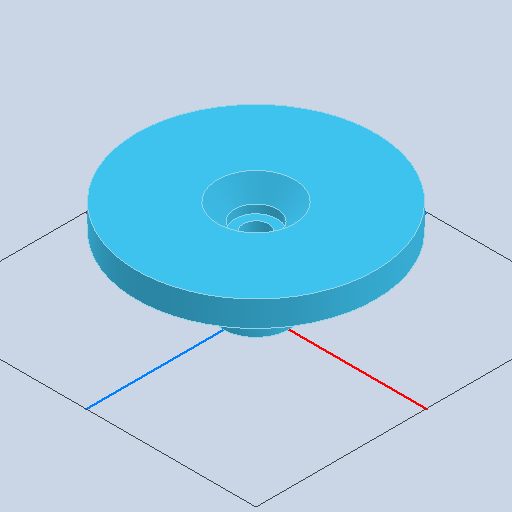
# Autodesk Inventor part: 000.005.002.003 - ВТУЛКА
Saved by Autodesk Inventor 2022 (Build 260153000, 153)
## iProperties
Created: 2022-11-19
Part Number: 000.005.002.003 - ВТУЛКА
Material: Пластик АБС
Document SubType Name: Modeling
Designer: Petrov Ivan
Density: 1.06 g/cm^3
Appearance: Бирюзовый
Mass: 2.20089 g
Surface Area: 17.8832 cm^2
Volume: 2.07631 cm^3
Author: Petrov Ivan
Autodesk Inventor part; units mm, degrees
ref_plane "YZ Plane" through (0, 0, 0) normal (1, 0, 0) x (0, 1, 0)
ref_plane "XZ Plane" through (0, 0, 0) normal (0, 1, 0) x (-1, 0, 0)
ref_plane "XY Plane" through (0, 0, 0) normal (0, 0, 1) x (1, 0, 0)
sketch "Эскиз1" plane through (0, 0, 0) normal (0, 1, 0) x (-1, 0, 0)
  circle A0 centre (0, 0) radius 3.9
  dimension "d0" = 7.8
  constraints: 1 centre point, 1 coincident
  measures "d0" diameter of A0
extrude "Выдавливание1" add sketch "Эскиз1" along normal blind 8.05
sketch "Эскиз2" plane through (0, 8.05, 0) normal (0, 1, 0) x (1, 0, 0)
  circle A0 centre (0, 0) radius 1.5
  dimension "d3" = 3
  constraints: 1 centre point, 1 coincident
  measures "d3" diameter of A0
extrude "Выдавливание2" cut sketch "Эскиз2" against normal blind 8.05
sketch "Эскиз3" plane through (0, 8.05, 0) normal (0, 1, 0) x (1, 0, 0)
  circle A0 centre (0, 0) radius 14
  circle A1 centre (0, 0) radius 1.5 projected
  dimension "d6" = 28
  constraints: 1 centre point, 1 coincident
  measures "d6" diameter of A0
extrude "Выдавливание3" add sketch "Эскиз3" along normal blind 3
sketch "Эскиз4" plane through (0, 11.05, 0) normal (0, 1, 0) x (1, 0, 0)
  circle A0 centre (0, 0) radius 2.5
  dimension "d9" = 5
  constraints: 1 centre point, 1 coincident
  measures "d9" diameter of A0
extrude "Выдавливание4" cut sketch "Эскиз4" against normal blind 3
chamfer "Фаска1" distance 2 angle 45 1 edges at (-2.5, 11.05, 0)
